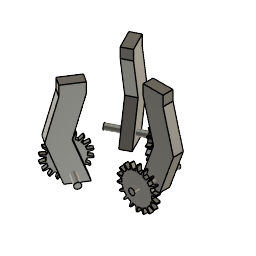
Fingers (Autodesk Fusion 360 design; units mm, degrees)
part number: 2026-03-20-16-49-33-089
Autodesk Fusion 360 part; units mm, degrees
sketch "Sketch2" plane through (0, 0, 0) normal (0, 0, 1) x (1, 0, 0)
  circle A0 centre (-139.7, 25.4) radius 19.05
  line L0 (-140.9543, 44.4087) -> (-140.4015, 50.7345)
  line L1 (-138.4228, 44.4071) -> (-138.9798, 50.7327)
  line L2 (-140.4015, 50.7345) -> (-138.9798, 50.7327)
  line L3 (-145.0006, 43.6977) -> (-147.6875, 49.4512)
  line L4 (-149.0241, 48.9668) -> (-147.6875, 49.4512)
  line L5 (-147.38, 42.8333) -> (-149.0241, 48.9668)
  line L6 (-150.9392, 40.7813) -> (-155.4318, 45.2689)
  line L7 (-156.5221, 44.3565) -> (-155.4318, 45.2689)
  line L8 (-152.8794, 39.1552) -> (-156.5221, 44.3565)
  line L9 (-155.5221, 36.0097) -> (-161.2786, 38.69)
  line L10 (-161.9911, 37.4598) -> (-161.2786, 38.69)
  line L11 (-156.7891, 33.8181) -> (-161.9911, 37.4598)
  line L12 (-158.1966, 29.9584) -> (-164.5227, 30.5082)
  line L13 (-164.7715, 29.1085) -> (-164.5227, 30.5082)
  line L14 (-158.6377, 27.4656) -> (-164.7715, 29.1085)
  line L15 (-158.6402, 23.3572) -> (-164.7729, 21.7103)
  line L16 (-164.5279, 20.3099) -> (-164.7729, 21.7103)
  line L17 (-158.2021, 20.8639) -> (-164.5279, 20.3099)
  line L18 (-156.7993, 17.0025) -> (-161.9988, 13.3574)
  line L19 (-161.2896, 12.1252) -> (-161.9988, 13.3574)
  line L20 (-155.5348, 14.8094) -> (-161.2896, 12.1252)
  line L21 (-152.896, 11.6607) -> (-156.5352, 6.457)
  line L22 (-155.4474, 5.5417) -> (-156.5352, 6.457)
  line L23 (-150.9577, 10.0323) -> (-155.4474, 5.5417)
  line L24 (-147.401, 7.976) -> (-149.041, 1.8414)
  line L25 (-147.7058, 1.3534) -> (-149.041, 1.8414)
  line L26 (-145.0227, 7.1087) -> (-147.7058, 1.3534)
  line L27 (-140.9772, 6.3929) -> (-140.4202, 0.0673)
  line L28 (-138.9985, 0.0655) -> (-140.4202, 0.0673)
  line L29 (-138.4457, 6.3913) -> (-138.9985, 0.0655)
  line L30 (-134.3994, 7.1023) -> (-131.7125, 1.3488)
  line L31 (-130.3759, 1.8332) -> (-131.7125, 1.3488)
  line L32 (-132.02, 7.9667) -> (-130.3759, 1.8332)
  line L33 (-128.4608, 10.0187) -> (-123.9682, 5.5311)
  line L34 (-122.8779, 6.4435) -> (-123.9682, 5.5311)
  line L35 (-126.5206, 11.6448) -> (-122.8779, 6.4435)
  line L36 (-123.8779, 14.7903) -> (-118.1214, 12.11)
  line L37 (-117.4089, 13.3402) -> (-118.1214, 12.11)
  line L38 (-122.6109, 16.9819) -> (-117.4089, 13.3402)
  line L39 (-121.2034, 20.8416) -> (-114.8773, 20.2918)
  line L40 (-114.6285, 21.6915) -> (-114.8773, 20.2918)
  line L41 (-120.7623, 23.3344) -> (-114.6285, 21.6915)
  line L42 (-120.7598, 27.4428) -> (-114.6272, 29.0897)
  line L43 (-114.8722, 30.4901) -> (-114.6272, 29.0897)
  line L44 (-121.1979, 29.9361) -> (-114.8722, 30.4901)
  line L45 (-122.6007, 33.7975) -> (-117.4012, 37.4426)
  line L46 (-118.1104, 38.6748) -> (-117.4012, 37.4426)
  line L47 (-123.8652, 35.9906) -> (-118.1104, 38.6748)
  line L48 (-126.5041, 39.1393) -> (-122.8648, 44.343)
  line L49 (-123.9526, 45.2583) -> (-122.8648, 44.343)
  line L50 (-128.4423, 40.7677) -> (-123.9526, 45.2583)
  line L51 (-131.999, 42.824) -> (-130.359, 48.9586)
  line L52 (-131.6942, 49.4466) -> (-130.359, 48.9586)
  line L53 (-134.3773, 43.6913) -> (-131.6942, 49.4466)
  dimension "d14" = 38.1
  dimension "d15" = 6.35
  dimension "d16" = 6.35
  dimension "d18" = 360
  constraint coincident A0 L0.start
  constraint coincident A0 L1.start
  measures "d14" diameter of A0
  measures "d15" distance of L0.start L0.end
  measures "d16" distance of L1.start L1.end
extrude "Extrude3" add sketch "Sketch2" along normal blind 5.08 makes body 1
sketch "Sketch3" plane through (0, 0, 0) normal (0, 0, 1) x (1, 0, 0)
  line L0 (0, 0) -> (17.3334, 47.7514)
  line L1 (-25.4, 0) -> (-7.9907, 47.7237)
  line L2 (17.3334, 47.7514) -> (4.2196, 96.8296)
  line L3 (-7.9907, 47.7237) -> (-21.1192, 96.798)
  line L4 (-21.1192, 96.798) -> (4.2196, 96.8296)
  line L5 (-25.4, 0) -> (0, 0)
  dimension "d21" = 50.8
  dimension "d22" = 50.8
  dimension "d23" = 50.8
  dimension "d24" = 50.8
  constraint coincident L0.start L5.end
  constraint horizontal L5
  measures "d21" distance of L0.start L0.end
  measures "d22" distance of L1.start L1.end
  measures "d23" distance of L0.end L2.end
  measures "d24" distance of L1.end L3.end
extrude "Extrude4" add sketch "Sketch3" along normal blind 12.7 separate body makes body 2
move_body "Move2" bodies 1 to x (1, 0, 0) y (0, 1, 0) z (0, 0, 1) at (130.81, -15.24, 12.7)
sketch "Sketch4" plane through (0, 0, 17.78) normal (0, 0, 1) x (-1, 0, 0)
  line L0 (7.6128, -29.1671) -> (8.1698, -35.4927)
  line L1 (8.1698, -35.4927) -> (9.5915, -35.4945)
  line L2 (9.5915, -35.4945) -> (10.1443, -29.1687)
  arc A0 (10.1443, -29.1687) -> (14.1906, -28.4577) centre (8.89, -10.16) ccw
  line L3 (14.1906, -28.4577) -> (16.8775, -34.2112)
  line L4 (16.8775, -34.2112) -> (18.2141, -33.7268)
  line L5 (18.2141, -33.7268) -> (16.57, -27.5933)
  arc A1 (16.57, -27.5933) -> (20.1292, -25.5413) centre (8.89, -10.16) ccw
  line L6 (20.1292, -25.5413) -> (24.6218, -30.0289)
  line L7 (24.6218, -30.0289) -> (25.7121, -29.1165)
  line L8 (25.7121, -29.1165) -> (22.0694, -23.9152)
  arc A2 (22.0694, -23.9152) -> (24.7121, -20.7697) centre (8.89, -10.16) ccw
  line L9 (24.7121, -20.7697) -> (30.4686, -23.45)
  line L10 (30.4686, -23.45) -> (31.1811, -22.2198)
  line L11 (31.1811, -22.2198) -> (25.9791, -18.5781)
  arc A3 (25.9791, -18.5781) -> (27.3866, -14.7184) centre (8.89, -10.16) ccw
  line L12 (27.3866, -14.7184) -> (33.7127, -15.2682)
  line L13 (33.7127, -15.2682) -> (33.9615, -13.8685)
  line L14 (33.9615, -13.8685) -> (27.8277, -12.2256)
  arc A4 (27.8277, -12.2256) -> (27.8302, -8.1172) centre (8.89, -10.16) ccw
  line L15 (27.8302, -8.1172) -> (33.9629, -6.4703)
  line L16 (33.9629, -6.4703) -> (33.7179, -5.0699)
  line L17 (33.7179, -5.0699) -> (27.3921, -5.6239)
  arc A5 (27.3921, -5.6239) -> (25.9893, -1.7625) centre (8.89, -10.16) ccw
  line L18 (25.9893, -1.7625) -> (31.1888, 1.8826)
  line L19 (31.1888, 1.8826) -> (30.4796, 3.1148)
  line L20 (30.4796, 3.1148) -> (24.7248, 0.4306)
  arc A6 (24.7248, 0.4306) -> (22.086, 3.5793) centre (8.89, -10.16) ccw
  line L21 (22.086, 3.5793) -> (25.7252, 8.783)
  line L22 (25.7252, 8.783) -> (24.6374, 9.6983)
  line L23 (24.6374, 9.6983) -> (20.1477, 5.2077)
  arc A7 (20.1477, 5.2077) -> (16.591, 7.264) centre (8.89, -10.16) ccw
  line L24 (16.591, 7.264) -> (18.231, 13.3986)
  line L25 (18.231, 13.3986) -> (16.8958, 13.8866)
  line L26 (16.8958, 13.8866) -> (14.2127, 8.1313)
  arc A8 (14.2127, 8.1313) -> (10.1672, 8.8471) centre (8.89, -10.16) ccw
  line L27 (10.1672, 8.8471) -> (9.6102, 15.1727)
  line L28 (9.6102, 15.1727) -> (8.1885, 15.1745)
  line L29 (8.1885, 15.1745) -> (7.6357, 8.8487)
  arc A9 (7.6357, 8.8487) -> (3.5894, 8.1377) centre (8.89, -10.16) ccw
  line L30 (3.5894, 8.1377) -> (0.9025, 13.8912)
  line L31 (0.9025, 13.8912) -> (-0.4341, 13.4068)
  line L32 (-0.4341, 13.4068) -> (1.21, 7.2733)
  arc A10 (1.21, 7.2733) -> (-2.3492, 5.2213) centre (8.89, -10.16) ccw
  line L33 (-2.3492, 5.2213) -> (-6.8418, 9.7089)
  line L34 (-6.8418, 9.7089) -> (-7.9321, 8.7965)
  line L35 (-7.9321, 8.7965) -> (-4.2894, 3.5952)
  arc A11 (-4.2894, 3.5952) -> (-6.9321, 0.4497) centre (8.89, -10.16) ccw
  line L36 (-6.9321, 0.4497) -> (-12.6886, 3.13)
  line L37 (-12.6886, 3.13) -> (-13.4011, 1.8998)
  line L38 (-13.4011, 1.8998) -> (-8.1991, -1.7419)
  arc A12 (-8.1991, -1.7419) -> (-9.6066, -5.6016) centre (8.89, -10.16) ccw
  line L39 (-9.6066, -5.6016) -> (-15.9327, -5.0518)
  line L40 (-15.9327, -5.0518) -> (-16.1815, -6.4515)
  line L41 (-16.1815, -6.4515) -> (-10.0477, -8.0944)
  arc A13 (-10.0477, -8.0944) -> (-10.0502, -12.2028) centre (8.89, -10.16) ccw
  line L42 (-10.0502, -12.2028) -> (-16.1828, -13.8497)
  line L43 (-16.1828, -13.8497) -> (-15.9378, -15.2501)
  line L44 (-15.9378, -15.2501) -> (-9.6121, -14.6961)
  arc A14 (-9.6121, -14.6961) -> (-8.2093, -18.5575) centre (8.89, -10.16) ccw
  line L45 (-8.2093, -18.5575) -> (-13.4088, -22.2026)
  line L46 (-13.4088, -22.2026) -> (-12.6996, -23.4348)
  line L47 (-12.6996, -23.4348) -> (-6.9448, -20.7506)
  arc A15 (-6.9448, -20.7506) -> (-4.3059, -23.8993) centre (8.89, -10.16) ccw
  line L48 (-4.3059, -23.8993) -> (-7.9452, -29.103)
  line L49 (-7.9452, -29.103) -> (-6.8574, -30.0183)
  line L50 (-6.8574, -30.0183) -> (-2.3677, -25.5277)
  arc A16 (-2.3677, -25.5277) -> (1.189, -27.584) centre (8.89, -10.16) ccw
  line L51 (1.189, -27.584) -> (-0.451, -33.7186)
  line L52 (-0.451, -33.7186) -> (0.8842, -34.2066)
  line L53 (0.8842, -34.2066) -> (3.5673, -28.4513)
  arc A17 (3.5673, -28.4513) -> (7.6128, -29.1671) centre (8.89, -10.16) ccw
  circle A18 centre (8.89, -10.16) radius 3.81
  dimension "d27" = 7.62
  constraint concentric A0 A18
  measures "d27" diameter of A18
extrude "Extrude5" add sketch "Sketch4" along normal mid plane 58.42 separate body contours A18 makes body 3
move_body "Move3" bodies 3 to x (1, 0, 0) y (0, 1, 0) z (0, 0, 1) at (0, 0, -7.62)
copy_body "CopyPasteBodies1" bodies 2 makes body 4
move_body "Move4" bodies 4 to x (1, 0, 0) y (0, 1, 0) z (0, 0, 1) at (-88.9, 0, 0)
copy_body "CopyPasteBodies2" bodies 3 makes body 5
move_body "Move5" bodies 5 to x (1, 0, 0) y (0, 1, 0) z (0, 0, 1) at (-88.9, 0, 0)
copy_body "CopyPasteBodies3" bodies 1 makes body 6
move_body "Move6" bodies 6 to x (1, 0, 0) y (0, 1, 0) z (0, 0, 1) at (-88.9, 0, 0)
copy_body "CopyPasteBodies4" bodies 4 6 5 makes body 7 makes body 8 makes body 9
move_body "Move7" bodies 7 8 9 to x (1, 0, 0) y (0, 1, 0) z (0, 0, 1) at (-88.9, 0, 0)
move_body "Move8" bodies 7 9 8 to x (1, 0, 0) y (0, 0, 1) z (0, -1, 0) at (0, 61.1148, -35.7148)
move_body "Move9" bodies 4 6 5 to x (1, 0, 0) y (0, 0, 1) z (0, -1, 0) at (0, 61.1148, -35.7148)
move_body "Move10" bodies 2 1 3 to x (1, 0, 0) y (0, 0, 1) z (0, -1, 0) at (0, 61.1148, -35.7148)
move_body "Move12" bodies 7 9 8 to x (-0.499998, -0.866025, -0.001867) y (0.866025, -0.5, 0.001078) z (-0.001867, -0.001078, 0.999998) at (-232.0022, -105.7721, 54.0724)
move_body "Move13" bodies 2 3 1 to x (1, 0, 0) y (0, 1, 0) z (0, 0, 1) at (13.057, 0, 35.7928)
move_body "Move14" bodies 7 8 9 to x (1, 0, 0) y (0, 1, 0) z (0, 0, 1) at (0.0119, -0.0068, -12.7)
move_body "Move15" bodies 4 5 6 to x (-0.499998, 0.866025, -0.001867) y (-0.866025, -0.5, -0.001078) z (-0.001867, 0.001078, 0.999998) at (-79.3477, 216.7581, 35.0807)
move_body "Move16" bodies 7 9 8 to x (0.996195, 0.087156, -0.000005) y (-0.087156, 0.996195, -0.000108) z (-0.000005, 0.000108, 1) at (52.7816, -0.8822, 0.0657)
move_body "Move17" bodies 4 5 6 to x (1, 0, 0) y (0, 1, 0) z (0, 0, 1) at (35.5478, -23.4706, 0.0443)
move_body "Move18" bodies 7 9 8 to x (1, 0, 0) y (0, 1, 0) z (0, 0, 1) at (0, 6.35, 0)
move_body "Move19" bodies 7 9 8 to x (0.996195, -0.087156, -0.000005) y (0.087156, 0.996195, 0.000108) z (-0.000005, -0.000108, 1) at (-2.3742, -3.4539, -0.003)
move_body "Move20" bodies 7 8 9 to x (1, 0, 0) y (0, 1, 0) z (0, 0, 1) at (-5.08, -5.08, -0.0063)
move_body "Move21" bodies 7 8 9 to x (0.996195, 0.087156, -0.000005) y (-0.087156, 0.996195, -0.000108) z (-0.000005, 0.000108, 1) at (-3.4779, -1.0089, -0.0043)
move_body "Move22" bodies 7 8 9 to x (0.984808, -0.173648, -0.000019) y (0.173648, 0.984808, 0.000216) z (-0.000019, -0.000216, 1) at (-8.5106, -13.6864, -0.0106)
move_body "Move23" bodies 7 8 9 to x (1, 0, 0) y (0, 1, 0) z (0, 0, 1) at (-5.08, -5.08, -0.0063)
move_body "Move24" bodies 7 9 8 to x (1, 0, 0) y (0, 1, 0) z (0, 0, 1) at (2.54, 2.54, 0.0032)
move_body "Move25" bodies 7 8 9 to x (1, 0, 0) y (0, 1, 0) z (0, 0, 1) at (0.0053, -0.0037, -6.35)
move_body "Move26" bodies 4 5 6 to x (1, 0, 0) y (0, 1, 0) z (0, 0, 1) at (-20.32, 20.32, -0.0253)
move_body "Move27" bodies 4 5 6 to x (1, 0, 0) y (0, 1, 0) z (0, 0, 1) at (2.54, -5.08, 0.0032)
move_body "Move28" bodies 4 5 6 to x (1, 0, 0) y (0, 1, 0) z (0, 0, 1) at (-5.08, -5.08, -0.0063)
move_body "Move29" bodies 4 5 6 to x (0.99863, -0.052336, -0.000002) y (0.052336, 0.99863, 0.000065) z (-0.000002, -0.000065, 1) at (-4.8953, -3.2973, -0.0061)
move_body "Move30" bodies 4 5 6 to x (1, 0, 0) y (0, 1, 0) z (0, 0, 1) at (1.1152, -2.1872, -0.6512)
move_body "Move31" bodies 1 to x (1, 0, 0) y (0, 1, 0) z (0, 0, 1) at (0, -15.24, 0)
move_body "Move32" bodies 8 to x (1, 0, 0) y (0, 1, 0) z (0, 0, 1) at (-12.4839, 8.7413, -0.0155)
move_body "Move33" bodies 6 to x (1, 0, 0) y (0, 1, 0) z (0, 0, 1) at (13.5789, 6.9188, 0.0169)
extrude "Extrude6" add 1 faces at (0.3841, 52.6481, 96.8866) along direction (-0.001245, 0, 0.999999) blind 12.7 on bodies 2 bodies 2
extrude "Extrude7" add 1 faces at (-54.4878, 9.9242, 96.5742) along direction (-0.001245, 0, 0.999999) blind 12.7 on bodies 7 bodies 7
extrude "Extrude8" add 1 faces at (-60.6085, 86.8346, 95.6716) along direction (-0.001245, 0, 0.999999) blind 12.7 on bodies 4 bodies 4
move_body "Move34" bodies 7 9 8 to x (0.996195, 0.087156, -0.000005) y (-0.087156, 0.996195, -0.000108) z (-0.000005, 0.000108, 1) at (0.4466, 5.1299, 0.0006)
move_body "Move35" bodies 7 9 8 to x (0.99863, -0.052336, -0.000002) y (0.052336, 0.99863, 0.000065) z (-0.000002, -0.000065, 1) at (-0.4821, -3.0524, -0.0006)
